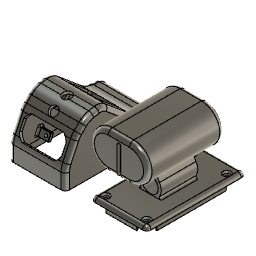
Boitier_CanneASon (Autodesk Fusion 360 design; units mm, degrees)
Autodesk Fusion 360 part; units mm, degrees
sketch "Sketch1" plane through (0, 0, 0) normal (1, 0, 0) x (0, 1, 0)
  line L0 (0, 0) -> (0, 12)
  line L1 (0, 12) -> (8.874983, 31.032464)
  line L2 (0, 12) -> (19, 12) construction
  line L3 (8.874983, 31.032464) -> (18.067372, 40.224852)
  line L4 (8.874983, 31.032464) -> (18.029747, 31.032464) construction
  line L5 (18.067372, 40.224852) -> (30.869872, 42.482278)
  line L6 (18.067372, 40.224852) -> (25.100815, 40.224852) construction
  line L7 (0, 0) -> (80, 0)
  line L8 (30.869872, 42.482278) -> (32.826168, 42.066455)
  line L9 (30.869872, 42.482278) -> (38.024636, 42.482278) construction
  line L10 (32.826168, 42.066455) -> (59.637723, 19.568888)
  line L11 (32.826168, 42.066455) -> (72.849817, 42.066455) construction
  line L12 (59.637723, 19.568888) -> (74.582285, 17.593812)
  line L13 (74.582285, 17.593812) -> (80, 0)
  dimension "d1" = 12
  dimension "d2" = 65
  dimension "d3" = 21
  dimension "d4" = 13
  dimension "d5" = 45
  dimension "d6" = 13
  dimension "d7" = 10
  dimension "d8" = 80
  dimension "d16" = 2
  dimension "d17" = 12
  dimension "d18" = 40
  dimension "d19" = 35
  constraint coincident L0.start L7.start
  constraint vertical L0
  constraint horizontal L2
  constraint horizontal L4
  constraint horizontal L6
  constraint perpendicular L0 L7
  constraint horizontal L9
  constraint horizontal L11
  measures "d1" distance of L0.start L0.end
  measures "d2" angle of L1 L2
  measures "d5" angle of L3 L4
  measures "d7" angle of L5 L6
  measures "d8" distance of L0.start L7.end
  measures "d17" angle of L8 L9
  measures "d18" angle of L10 L11
extrude "Extrude2" add sketch "Sketch1" along normal blind 46 contours L0 L1 L3 L5 L7 L8 L10 L12 L13 picked at (46.545908, 6.522963) makes body 1
sketch "Sketch2" plane through (0, -11.07874, 11.07874) normal (0, -0.707107, 0.707107) x (1, 0, 0)
  line L0 (0, 41.218826) -> (0, 28.218826)
  line L1 (0, 28.218826) -> (46, 28.218826)
  line L2 (46, 28.218826) -> (46, 41.218826)
  line L3 (46, 41.218826) -> (0, 41.218826)
  circle A0 centre (23, 34.718826) radius 3.75
  dimension "d26" = 7.5
  measures "d26" diameter of A0
shell "Shell2" thickness 2.5 removed faces 1 at (15.333333, 26.666667, 0) on bodies 1
extrude "Extrude3" cut sketch "Sketch2" against normal blind 15 contours A0 picked at (22.721849, 35.827351) bodies 1
sketch "Sketch3" plane through (0, -6.334057, 35.922221) normal (0, -0.173648, 0.984808) x (1, 0, 0)
  line L0 (0, 37.77786) -> (0, 24.77786)
  line L1 (0, 24.77786) -> (46, 24.77786)
  line L2 (46, 24.77786) -> (46, 37.77786)
  line L3 (46, 37.77786) -> (0, 37.77786)
  circle A0 centre (23, 31.27786) radius 3.75
  dimension "d30" = 7.5
  measures "d30" diameter of A0
extrude "Extrude4" cut sketch "Sketch3" against normal blind 6 contours A0 picked at (22.721849, 32.386384) bodies 1
sketch "Sketch7" plane through (0, 34.276667, 40.849341) normal (0, 0.642788, 0.766044) x (-1, 0, 0)
  line L0 (0, -33.106508) -> (0, 1.893492)
  line L1 (0, 1.893492) -> (-46, 1.893492)
  line L2 (-46, 1.893492) -> (-46, -33.106508)
  line L3 (-33.1, -28.248154) -> (-12.9, -28.248154)
  line L4 (-10.9, -26.248154) -> (-10.9, -6.048154)
  line L5 (-12.9, -4.048154) -> (-33.1, -4.048154)
  line L6 (-35.1, -6.048154) -> (-35.1, -26.248154)
  arc A0 (-33.1, -4.048154) -> (-35.1, -6.048154) centre (-33.1, -6.048154) ccw
  arc A1 (-35.1, -26.248154) -> (-33.1, -28.248154) centre (-33.1, -26.248154) ccw
  arc A2 (-12.9, -28.248154) -> (-10.9, -26.248154) centre (-12.9, -26.248154) ccw
  arc A3 (-10.9, -6.048154) -> (-12.9, -4.048154) centre (-12.9, -6.048154) ccw
  line L7 (-46, -33.106508) -> (0, -33.106508)
  point P0 (-35.1, -28.248154)
  point P1 (-10.9, -28.248154)
  point P2 (-35.1, -4.048154)
  dimension "d42" = 24.2
  dimension "d43" = 24.2
  dimension "d44" = 2
  constraint horizontal L3
  constraint vertical L4
  constraint horizontal L5
  constraint vertical L6
  constraint tangent L5 A0
  constraint tangent L6 A0
  constraint tangent L3 A1
  constraint tangent L6 A1
  constraint equal A0 A1
  constraint tangent L3 A2
  constraint tangent L4 A2
  constraint equal A0 A2
  constraint tangent L4 A3
  constraint tangent L5 A3
  constraint equal A0 A3
  measures "d44" radius of A0
extrude "Extrude7" add sketch "Sketch7" against normal blind 14 separate body contours L3 L4 L5 L6 A0 A1 A2 A3 picked at (-19.633333, -13.448154) makes body 2
shell "Shell3" thickness 3 outward yes removed faces 1 at (26.366667, 44.578551, 32.205034) on bodies 2
extrude "Extrude8" cut sketch "Sketch7" against normal blind 14 contours L3 L4 L5 L6 A0 A1 A2 A3 picked at (-19.633333, -13.448154) bodies 1
combine "Combine1" operation add target body 1 tool bodies 2
sketch "Sketch8" plane through (0, -4.596267, 2.143274) normal (0, -0.906308, 0.422618) x (1, 0, 0)
  line L0 (0, 31.875693) -> (0, 10.875693)
  line L1 (0, 10.875693) -> (46, 10.875693)
  line L2 (46, 10.875693) -> (46, 31.875693)
  line L3 (46, 31.875693) -> (0, 31.875693)
  line L4 (5.6, 12.175693) -> (40.4, 12.175693)
  line L5 (40.4, 12.175693) -> (40.4, 30.575693)
  line L6 (40.4, 30.575693) -> (5.6, 30.575693)
  line L7 (5.6, 30.575693) -> (5.6, 12.175693)
  line L8 (5.6, 12.175693) -> (5.6, 17.175693)
  line L9 (5.6, 21.375693) -> (15.6, 21.375693)
  circle A0 centre (15.6, 21.375693) radius 10.846197
  line L10 (40.4, 21.375693) -> (30.4, 21.375693)
  line L11 (40.4, 30.575693) -> (40.4, 25.575693)
  circle A1 centre (30.4, 21.375693) radius 10.846197
  dimension "d58" = 34.8
  dimension "d59" = 18.4
  dimension "d61" = 5
  dimension "d62" = 10
  dimension "d63" = 10
  dimension "d64" = 5
  constraint horizontal L4
  constraint vertical L5
  constraint horizontal L6
  constraint vertical L7
  constraint perpendicular L4 L8
  constraint perpendicular L7 L9
  constraint perpendicular L5 L10
  constraint perpendicular L6 L11
extrude "Extrude9" cut sketch "Sketch8" against normal blind 11 contours L4 L6 L7 A0 A1 | L6 A0 A1 | L4 A0 A1 | L4 L5 L6 A0 A1 | A0 A1 picked at (10.458254, 19.308066) picked at (22.825261, 30.046675) picked at (23.174739, 12.704712) picked at (35.518079, 19.084776) picked at (21.871346, 21.375693) bodies 1
sketch "Sketch12" plane through (0, 14.436197, -6.731709) normal (0, 0.906308, -0.422618) x (-1, 0, 0)
  line L0 (-36.144563, 30.575693) -> (-40.4, 30.575693)
  line L1 (-40.4, 30.575693) -> (-40.4, 25.575693)
  arc A0 (-36.144563, 30.575693) -> (-40.4, 25.575693) centre (-30.4, 21.375693) ccw
  line L2 (-34.000001, 30.125693) -> (-44.000001, 30.125693)
  line L3 (-44.000001, 30.125693) -> (-44.000001, 24.125693)
  line L4 (-44.000001, 24.125693) -> (-34.000001, 24.125693)
  line L5 (-34.000001, 24.125693) -> (-34.000001, 30.125693)
  circle A1 centre (-37.000001, 27.125693) radius 1.2
  dimension "d95" = 10
  dimension "d96" = 6
  dimension "d97" = 2.4
  constraint horizontal L2
  constraint vertical L3
  constraint horizontal L4
  constraint vertical L5
  measures "d97" diameter of A1
extrude "Extrude12" add sketch "Sketch12" along normal blind 2.5 separate body contours L1 A0 L2 L3 L4 L5 | L1 A0 L2 picked at (-42.8, 26.609027) picked at (-39.081529, 29.134109) makes body 3
sketch "Sketch13" plane through (0, 14.436197, -6.731709) normal (0, 0.906308, -0.422618) x (-1, 0, 0)
  line L0 (-9.855437, 12.175693) -> (-5.6, 12.175693)
  line L1 (-5.6, 12.175693) -> (-5.6, 17.175693)
  arc A0 (-9.855437, 12.175693) -> (-5.6, 17.175693) centre (-15.6, 21.375693) ccw
  line L2 (-12, 12.625693) -> (-2.5, 12.625693)
  line L3 (-2.5, 12.625693) -> (-2.5, 18.625693)
  line L4 (-2.5, 18.625693) -> (-12, 18.625693)
  line L5 (-12, 18.625693) -> (-12, 12.625693)
  circle A1 centre (-9, 15.625693) radius 1.2
  dimension "d104" = 6
  dimension "d105" = 2.4
  constraint horizontal L2
  constraint vertical L3
  constraint horizontal L4
  constraint vertical L5
  measures "d105" diameter of A1
extrude "Extrude13" add sketch "Sketch13" along normal blind 2.5 separate body contours L1 A0 L2 L3 L4 L5 | L1 A0 L2 picked at (-3.533333, 16.14236) picked at (-6.918471, 13.617278) makes body 4
fillet "Fillet8" radius 0.3 16 edges at (39.000001, 24.632155, 15.133595) (39.000001, 27.167865, 20.571441) (39.000001, 29.433635, 19.514896) (39.000001, 26.897925, 14.077049) (34.000001, 28.30075, 20.043169) (34.000001, 25.76504, 14.605322) (34.000001, 25.90001, 17.852518) (34.000001, 28.16578, 16.795972) (7.25, 22.307755, 10.148902) (7.25, 19.772045, 4.711055) (7.25, 24.573525, 9.092356) (7.25, 22.037815, 3.654509) (12, 23.44064, 9.620629) (12, 21.0399, 7.429978) (12, 20.90493, 4.182782) (12, 23.30567, 6.373433) on bodies 3 4
combine "Combine2" operation add target body 1 tool bodies 4 3
fillet "Fillet9" radius 1.5 8 edges at (2.5, 20.90493, 4.182782) (2.5, 19.888816, 4.753556) (2.5, 21.0399, 7.429978) (2.5, 22.350256, 10.032132) (2.5, 23.44064, 9.620629) (2.5, 24.456754, 9.049855) (2.5, 23.30567, 6.373433) (2.5, 21.995314, 3.77128) on bodies 1
fillet "Fillet10" radius 1.5 8 edges at (43.5, 28.16578, 16.795972) (43.5, 29.316865, 19.472395) (43.5, 28.30075, 20.043169) (43.5, 27.210366, 20.454671) (43.5, 25.90001, 17.852518) (43.5, 24.748926, 15.176095) (43.5, 25.76504, 14.605322) (43.5, 26.855424, 14.193819) on bodies 1
sketch "Sketch14" plane through (0, 25.277641, 30.124719) normal (0, 0.642788, 0.766044) x (-1, 0, 0)
  arc A0 (-10.9, -6.048154) -> (-12.9, -4.048154) centre (-12.9, -6.048154) ccw
  line L0 (-12.9, -4.048154) -> (-33.1, -4.048154)
  arc A1 (-33.1, -4.048154) -> (-35.1, -6.048154) centre (-33.1, -6.048154) ccw
  line L1 (-35.1, -6.048154) -> (-35.1, -26.248154)
  arc A2 (-35.1, -26.248154) -> (-33.1, -28.248154) centre (-33.1, -26.248154) ccw
  line L2 (-33.1, -28.248154) -> (-12.9, -28.248154)
  arc A3 (-12.9, -28.248154) -> (-10.9, -26.248154) centre (-12.9, -26.248154) ccw
  line L3 (-10.9, -26.248154) -> (-10.9, -6.048154)
  line L4 (-32.5, -28.248154) -> (-13.5, -28.248154)
  line L5 (-13.5, -28.248154) -> (-13.5, -3.748154)
  line L6 (-13.5, -3.748154) -> (-32.5, -3.748154)
  line L7 (-32.5, -3.748154) -> (-32.5, -28.248154)
  dimension "d115" = 19
  constraint horizontal L4
  constraint vertical L5
  constraint horizontal L6
  constraint vertical L7
extrude "Extrude14" cut sketch "Sketch14" against normal blind 2 contours L0 L2 L4 L5 L7 picked at (-26.166667, -12.11482) bodies 1
extrude "Extrude15" cut 1 faces at (26.166667, 33.272556, 20.805373) along direction (0, -0.64278761, -0.76604444) blind 1 on bodies 1 bodies 1
sketch "Sketch15" plane through (0, 23.937475, -20.085926) normal (0, 0.766044, -0.642788) x (-1, 0, 0)
  line L0 (-12.9, 50.825028) -> (-33.1, 50.825028)
  line L1 (-33.1, 50.825028) -> (-33.1, 36.325028)
  line L2 (-33.1, 36.325028) -> (-12.9, 36.325028)
  line L3 (-12.9, 36.325028) -> (-12.9, 50.825028)
  line L4 (-33.1, 36.325028) -> (-29.35, 36.325028)
  line L5 (-29.35, 36.325028) -> (-16.35, 36.325028)
  line L6 (-16.35, 36.325028) -> (-16.35, 50.825028)
  line L7 (-16.35, 50.825028) -> (-29.35, 50.825028)
  line L8 (-29.35, 50.825028) -> (-29.35, 36.325028)
  dimension "d120" = 3.75
  dimension "d121" = 13
  dimension "d122" = 14.5
  constraint perpendicular L1 L4
  constraint horizontal L5
  constraint vertical L6
  constraint horizontal L7
  constraint vertical L8
extrude "Extrude16" cut sketch "Sketch15" against normal blind 31 contours L0 L2 L5 L6 L7 L8 picked at (-20.683333, 41.158361) bodies 1
fillet "Fillet11" radius 2 4 edges at (29.35, 46.137686, 8.704841) (29.35, 25.301277, 26.188664) (16.35, 25.301277, 26.188664) (16.35, 46.137686, 8.704841) on bodies 1
sketch "Sketch20" plane through (43.5, 0, 0) normal (-1, 0, 0) x (0, -1, 0)
  line L0 (-77.384156, 0) -> (-2.5, 0)
  line L1 (-2.5, 0) -> (-2.5, 11.445763)
  line L2 (-2.5, 11.445763) -> (-10.954455, 29.576402)
  line L3 (-10.954455, 29.576402) -> (-19.277764, 37.89971)
  line L4 (-19.277764, 37.89971) -> (-30.825425, 39.935874)
  line L5 (-30.825425, 39.935874) -> (-31.696689, 39.750681)
  line L6 (-31.696689, 39.750681) -> (-58.58844, 17.185823)
  line L7 (-58.58844, 17.185823) -> (-72.664938, 15.32547)
  line L8 (-72.664938, 15.32547) -> (-77.384156, 0)
  line L9 (-28.384172, 13.715014) -> (-30.666311, 18.609076)
  arc A0 (-29.79567, 21.001143) -> (-30.666311, 18.609076) centre (-29.034957, 19.369789) ccw
  line L10 (-29.79567, 21.001143) -> (-28.073685, 21.804118)
  arc A1 (-25.681618, 20.933476) -> (-28.073685, 21.804118) centre (-27.312972, 20.172764) ccw
  line L11 (-25.681618, 20.933476) -> (-23.399479, 16.039414)
  arc A2 (-24.27012, 13.647348) -> (-23.399479, 16.039414) centre (-25.030833, 15.278702) ccw
  line L12 (-24.27012, 13.647348) -> (-25.992105, 12.844373)
  arc A3 (-28.384172, 13.715014) -> (-25.992105, 12.844373) centre (-26.752818, 14.475727) ccw
  line L13 (-71.626194, 13.560847) -> (-57.426194, 13.560847)
  line L14 (-57.426194, 13.560847) -> (-57.426194, 4.360847)
  line L15 (-57.426194, 4.360847) -> (-71.626194, 4.360847)
  line L16 (-71.626194, 4.360847) -> (-71.626194, 13.560847)
  dimension "d132" = 14.2
  dimension "d133" = 9.2
  constraint horizontal L13
  constraint vertical L14
  constraint horizontal L15
  constraint vertical L16
extrude "Extrude17" cut sketch "Sketch20" against normal blind 17 contours L13 L14 L15 L16 picked at (-66.892861, 10.494181) bodies 1
sketch "Sketch21" plane through (2.5, 0, 0) normal (1, 0, 0) x (0, 1, 0)
  line L0 (2.5, 0) -> (77.384156, 0)
  line L1 (77.384156, 0) -> (72.664938, 15.32547)
  line L2 (72.664938, 15.32547) -> (58.58844, 17.185823)
  line L3 (58.58844, 17.185823) -> (31.696689, 39.750681)
  line L4 (31.696689, 39.750681) -> (30.825425, 39.935874)
  line L5 (30.825425, 39.935874) -> (19.277764, 37.89971)
  line L6 (19.277764, 37.89971) -> (10.954455, 29.576402)
  line L7 (10.954455, 29.576402) -> (2.5, 11.445763)
  line L8 (2.5, 11.445763) -> (2.5, 0)
  line L9 (21.131995, 2.421833) -> (19.41001, 3.224808)
  arc A0 (18.539369, 5.616875) -> (19.41001, 3.224808) centre (20.170723, 4.856162) ccw
  line L10 (18.539369, 5.616875) -> (20.821508, 10.510937)
  arc A1 (23.213575, 11.381578) -> (20.821508, 10.510937) centre (22.452862, 9.750224) ccw
  line L11 (23.213575, 11.381578) -> (24.93556, 10.578603)
  arc A2 (25.806201, 8.186536) -> (24.93556, 10.578603) centre (24.174847, 8.947249) ccw
  line L12 (25.806201, 8.186536) -> (23.524062, 3.292474)
  arc A3 (21.131995, 2.421833) -> (23.524062, 3.292474) centre (21.892708, 4.053187) ccw
  line L13 (26, 0) -> (17, 0)
  line L14 (17, 0) -> (17, 4)
  line L15 (17, 4) -> (26, 4)
  line L16 (26, 4) -> (26, 0)
  dimension "d136" = 4
  constraint horizontal L13
  constraint vertical L14
  constraint horizontal L15
  constraint vertical L16
  constraint coincident L0 L13.start
  measures "d136" distance of L13.start L15.end
extrude "Extrude18" cut sketch "Sketch21" along normal blind 12 contours L0 L9 A0 L12 A3 L13 L14 L15 L16 | L9 A0 L12 A3 L15 picked at (21.626143, 0.751081) picked at (21.465331, 3.215547) bodies 1
sketch "Sketch23" plane through (46, 0, 0) normal (1, 0, 0) x (0, 1, 0)
  line L0 (57.426194, 4.360847) -> (57.426194, 13.560847)
  line L1 (57.426194, 13.560847) -> (71.626194, 13.560847)
  line L2 (71.626194, 13.560847) -> (71.626194, 4.360847)
  line L3 (71.626194, 4.360847) -> (57.426194, 4.360847)
  line L4 (0, 0) -> (80, 0)
  line L5 (80, 0) -> (74.582285, 17.593812)
  line L6 (74.582285, 17.593812) -> (59.637723, 19.568888)
  line L7 (59.637723, 19.568888) -> (32.826168, 42.066455)
  line L8 (32.826168, 42.066455) -> (30.869872, 42.482278)
  line L9 (30.869872, 42.482278) -> (18.067372, 40.224852)
  line L10 (18.067372, 40.224852) -> (8.874983, 31.032464)
  line L11 (8.874983, 31.032464) -> (0, 12)
  line L12 (0, 12) -> (0, 0)
  line L13 (0, 0) -> (0, -4)
  line L14 (0, -4) -> (97.000001, -4)
  line L15 (80, 0) -> (81.231732, -4)
  dimension "d143" = 4
  constraint coincident L4.start L12.end
  constraint perpendicular L4 L13
  constraint perpendicular L13 L14
  constraint coincident L4.end L5.start
  constraint parallel L5 L15
  measures "d143" distance of L4.start L13.end
extrude "Extrude20" add sketch "Sketch23" against normal blind 46 separate body contours L4 L13 L14 L15 picked at (53.743911, -2.666667) makes body 5
shell "Shell4" thickness 2.5 removed faces 2 at (30.666667, 27.077244, -4) at (30.666667, 26.666667, 0) on bodies 5
combine "Combine3" operation add target body 1 tool bodies 5
move_body "Move1" bodies 1 to x (1, 0, 0) y (0, 1, 0) z (0, 0, 1) at (0, 0, 4)
sketch "Sketch24" plane through (0, 0, 0) normal (0, 0, -1) x (1, 0, 0)
  line L0 (2.5, -2.5) -> (43.5, -2.5)
  line L1 (43.5, -2.5) -> (43.5, -78.615887)
  line L2 (43.5, -78.615887) -> (2.5, -78.615887)
  line L3 (2.5, -78.615887) -> (2.5, -2.5)
  line L4 (46, -81.231732) -> (46, 0)
  line L5 (46, 0) -> (0, 0)
  line L6 (0, 0) -> (0, -81.231732)
  line L7 (0, -81.231732) -> (46, -81.231732)
  line L8 (0, 0) -> (46, 0)
  line L9 (46, 0) -> (46, -81.231732)
  line L10 (46, -81.231732) -> (0, -81.231732)
  line L11 (0, -81.231732) -> (0, 0)
  constraint horizontal L8
  constraint vertical L9
  constraint horizontal L10
  constraint vertical L11
  constraint coincident L5.end L6.start
move_body "Move2" bodies 1 to x (1, 0, 0) y (0, 1, 0) z (0, 0, 1) at (-65, 0, 0)
extrude "Extrude21" add sketch "Sketch24" against normal blind 3 separate body contours L0 L1 L2 L3 | L4 L5 L6 L7 L8 L9 L10 L11 picked at (16.166667, -27.871962) picked at (29.833333, -80.359784) makes body 6
sketch "Sketch25" plane through (0, 0, 3) normal (0, 0, 1) x (-1, 0, 0)
  line L0 (-46, -81.231732) -> (0, -81.231732)
  line L1 (0, -81.231732) -> (0, 0)
  line L2 (0, 0) -> (-46, 0)
  line L3 (-46, 0) -> (-46, -81.231732)
  line L4 (-2.95, -69.1) -> (-2.05, -69.1)
  line L5 (-2.05, -69.1) -> (-2.05, -2.05)
  line L6 (-2.05, -2.05) -> (-43.95, -2.05)
  line L7 (-43.95, -2.05) -> (-43.95, -69.100001)
  line L8 (-43.95, -69.100001) -> (-43.05, -69.100001)
  line L9 (-43.05, -69.100001) -> (-43.05, -2.950001)
  line L10 (-43.05, -2.950001) -> (-2.95, -2.950001)
  line L11 (-2.95, -69.1) -> (-2.95, -2.950001)
  dimension "d151" = 0.9
  dimension "d152" = 67.05
  dimension "d153" = 41.9
  dimension "d154" = 67.050001
  dimension "d155" = 0.9
  dimension "d156" = 66.15
  dimension "d158" = 40.1
  constraint perpendicular L4 L5
  constraint perpendicular L3 L6
  constraint perpendicular L6 L7
  constraint perpendicular L7 L8
  constraint perpendicular L8 L9
  constraint perpendicular L9 L10
  constraint perpendicular L10 L11
  measures "d151" distance of L4.start L4.end
  measures "d152" distance of L4.end L5.end
  measures "d153" distance of L6.end L5.end
extrude "Extrude22" add sketch "Sketch25" along normal blind 5 contours L4 L5 L6 L7 L8 L9 L10 L11 picked at (-43.65, -24.700001) bodies 6
sketch "Sketch27" plane through (0, 0, 0) normal (0, 0, -1) x (1, 0, 0)
  line L0 (-62.5, -2.5) -> (-21.5, -2.5)
  line L1 (-21.5, -2.5) -> (-21.5, -78.615887)
  line L2 (-21.5, -78.615887) -> (-62.5, -78.615887)
  line L3 (-62.5, -78.615887) -> (-62.5, -2.5)
  line L4 (-19, -81.231732) -> (-19, 0)
  line L5 (-19, 0) -> (-65, 0)
  line L6 (-65, 0) -> (-65, -81.231732)
  line L7 (-65, -81.231732) -> (-19, -81.231732)
  line L8 (-63.05, -1.95) -> (-63.05, -74.1)
  line L9 (-63.05, -1.95) -> (-20.95, -1.95)
  line L10 (-20.95, -1.95) -> (-20.95, -74.1)
  line L11 (-20.95, -74.1) -> (-21.5, -74.1)
  line L12 (-21.5, -2.5) -> (-62.5, -2.5)
  line L13 (-63.05, -74.1) -> (-62.5, -74.1)
  line L14 (-62.5, -2.5) -> (-62.5, -74.1)
  dimension "d168" = 72.15
  dimension "d169" = 42.1
  dimension "d170" = 72.15
  constraint perpendicular L0 L8
  constraint perpendicular L4 L9
  constraint perpendicular L9 L10
  constraint coincident L1 L11.end
  constraint perpendicular L1 L11
  constraint coincident L0.end L1.start
  constraint coincident L0.start L3.end
  constraint coincident L3 L13.end
  constraint perpendicular L3 L13
  measures "d168" distance of L8.start L8.end
  measures "d169" distance of L8.start L9.end
  measures "d170" distance of L9.end L10.end
extrude "Extrude23" cut sketch "Sketch27" against normal blind 5.3 contours L0 L1 L3 L8 L9 L10 L11 L12 L13 L14 picked at (-21.133333, -26.183333) bodies 1
sketch "Sketch28" plane through (0, 0, 3) normal (0, 0, 1) x (-1, 0, 0)
  line L0 (-2.95, -69.1) -> (-2.95, -2.950001)
  line L1 (-2.95, -2.950001) -> (-43.05, -2.950001)
  line L2 (-43.05, -2.950001) -> (-43.05, -69.100001)
  line L3 (-43.95, -69.100001) -> (-43.95, -2.05)
  line L4 (-43.95, -2.05) -> (-2.05, -2.05)
  line L5 (-2.05, -2.05) -> (-2.05, -69.1)
  line L6 (-46, -81.231732) -> (0, -81.231732)
  line L7 (0, -81.231732) -> (0, 0)
  line L8 (0, 0) -> (-46, 0)
  line L9 (-46, 0) -> (-46, -81.231732)
  line L10 (-2.05, -2.05) -> (-10.05, -2.05)
  line L11 (-10.05, -2.05) -> (-10.05, -10.05)
  line L12 (-10.05, -10.05) -> (-2.05, -10.05)
  line L13 (-2.05, -10.05) -> (-2.05, -2.05)
  line L14 (-43.95, -2.05) -> (-35.95, -2.05)
  line L15 (-35.95, -2.05) -> (-35.95, -10.05)
  line L16 (-35.95, -10.05) -> (-43.95, -10.05)
  line L17 (-43.95, -10.05) -> (-43.95, -2.05)
  line L18 (-2.05, -69.1) -> (-2.95, -69.1)
  line L19 (-43.05, -69.100001) -> (-43.95, -69.100001)
  dimension "d174" = 8
  dimension "d175" = 8
  dimension "d176" = 8
  dimension "d177" = 8
  constraint horizontal L10
  constraint vertical L11
  constraint horizontal L12
  constraint vertical L13
  constraint coincident L4.end L5.start
  constraint horizontal L14
  constraint vertical L15
  constraint horizontal L16
  constraint vertical L17
  constraint coincident L3.end L4.start
  measures "d174" distance of L4.end L10.end
  measures "d175" distance of L4.end L12.end
  measures "d176" distance of L3.end L14.end
  measures "d177" distance of L3.end L16.end
extrude "Extrude24" add sketch "Sketch28" along normal blind 1 contours L0 L1 L11 L12 | L1 L2 L15 L16 picked at (-7.683333, -7.683334) picked at (-40.683333, -5.316667) bodies 6
sketch "Sketch29" plane through (0, 0, 0) normal (0, 0, -1) x (1, 0, 0)
  line L0 (-19, -81.231732) -> (-19, 0)
  line L1 (-19, 0) -> (-65, 0)
  line L2 (-65, 0) -> (-65, -81.231732)
  line L3 (-65, -81.231732) -> (-19, -81.231732)
  line L4 (-62.5, -74.1) -> (-63.05, -74.1)
  line L5 (-63.05, -74.1) -> (-63.05, -1.95)
  line L6 (-63.05, -1.95) -> (-20.95, -1.95)
  line L7 (-20.95, -1.95) -> (-20.95, -74.1)
  line L8 (-20.95, -74.1) -> (-21.5, -74.1)
  line L9 (-21.5, -74.1) -> (-21.5, -78.615887)
  line L10 (-21.5, -78.615887) -> (-62.5, -78.615887)
  line L11 (-62.5, -78.615887) -> (-62.5, -74.1)
  line L12 (-63.05, -1.95) -> (-54.95, -1.95)
  line L13 (-54.95, -1.95) -> (-54.95, -10.05)
  line L14 (-54.95, -10.05) -> (-63.05, -10.05)
  line L15 (-63.05, -10.05) -> (-63.05, -1.95)
  line L16 (-20.95, -1.95) -> (-29.05, -1.95)
  line L17 (-29.05, -1.95) -> (-29.05, -10.05)
  line L18 (-29.05, -10.05) -> (-20.95, -10.05)
  line L19 (-20.95, -10.05) -> (-20.95, -1.95)
  dimension "d180" = 8.1
  dimension "d181" = 8.1
  dimension "d182" = 8.1
  dimension "d183" = 8.1
  constraint horizontal L12
  constraint vertical L13
  constraint horizontal L14
  constraint vertical L15
  constraint coincident L5.end L6.start
  constraint horizontal L16
  constraint vertical L17
  constraint horizontal L18
  constraint vertical L19
  constraint coincident L6.end L7.start
  measures "d180" distance of L5.end L12.end
  measures "d181" distance of L5.end L14.end
  measures "d182" distance of L6.end L16.end
  measures "d183" distance of L6.end L18.end
extrude "Extrude25" add sketch "Sketch29" against normal blind 6 contours L5 L6 L12 L13 L14 L15 | L6 L7 L16 L17 L18 L19 picked at (-60.35, -4.65) picked at (-26.35, -4.65) bodies 1
extrude "Extrude26" cut sketch "Sketch29" against normal blind 1 contours L5 L6 L12 L13 L14 L15 | L6 L7 L16 L17 L18 L19 picked at (-60.35, -4.65) picked at (-26.35, -4.65) bodies 1
sketch "Sketch30" plane through (0, 0, 1) normal (0, 0, -1) x (1, 0, 0)
  line L0 (-63.05, -10.05) -> (-54.95, -10.05)
  line L1 (-54.95, -10.05) -> (-54.95, -1.95)
  line L2 (-54.95, -1.95) -> (-63.05, -1.95)
  line L3 (-63.05, -1.95) -> (-63.05, -10.05)
  line L4 (-63.05, -10.05) -> (-63.05, -67.55)
  line L5 (-63.05, -67.55) -> (-54.95, -67.55)
  line L6 (-54.95, -67.55) -> (-54.95, -76.15)
  line L7 (-54.95, -76.15) -> (-63.05, -76.15)
  line L8 (-63.05, -76.15) -> (-63.05, -67.55)
  line L9 (-20.95, -10.05) -> (-20.95, -67.55)
  line L10 (-20.95, -67.55) -> (-29.05, -67.55)
  line L11 (-29.05, -67.55) -> (-29.05, -76.15)
  line L12 (-29.05, -76.15) -> (-20.95, -76.15)
  line L13 (-20.95, -76.15) -> (-20.95, -67.55)
  dimension "d188" = 57.5
  dimension "d189" = 8.1
  dimension "d190" = 8.6
  dimension "d196" = 57.5
  dimension "d197" = 8.1
  dimension "d198" = 8.6
  constraint coincident L0.start L3.end
  constraint perpendicular L0 L4
  constraint horizontal L5
  constraint vertical L6
  constraint horizontal L7
  constraint vertical L8
  constraint vertical L9
  constraint horizontal L10
  constraint vertical L11
  constraint horizontal L12
  constraint vertical L13
  measures "d188" distance of L0.start L4.end
  measures "d189" distance of L4.end L5.end
  measures "d190" distance of L4.end L7.end
  measures "d196" distance of L9.start L9.end
  measures "d197" distance of L9.end L10.end
  measures "d198" distance of L9.end L12.end
extrude "Extrude28" add sketch "Sketch30" against normal blind 5 contours L5 L6 L7 L8 | L10 L11 L12 L13 picked at (-57.65, -70.416667) picked at (-26.35, -70.416667) bodies 1
extrude "Extrude29" cut 2 faces at (-21.316667, 74.1, 0.666667) (-62.866667, 74.1, 0.333333) along direction (0, 1, 0) blind 4 on bodies 1 bodies 1
sketch "Sketch31" plane through (0, 0, 8) normal (0, 0, 1) x (-1, 0, 0)
  line L0 (-2.05, -69.1) -> (-2.05, -2.05)
  line L1 (-2.05, -2.05) -> (-43.95, -2.05)
  line L2 (-43.95, -2.05) -> (-43.95, -69.100001)
  line L3 (-43.95, -69.100001) -> (-43.05, -69.100001)
  line L4 (-43.05, -69.100001) -> (-43.05, -2.950001)
  line L5 (-43.05, -2.950001) -> (-2.95, -2.950001)
  line L6 (-2.95, -2.950001) -> (-2.95, -69.1)
  line L7 (-2.95, -69.1) -> (-2.05, -69.1)
  line L8 (-2.05, -2.05) -> (-2.05, -10.35)
  line L9 (-2.05, -10.35) -> (-2.95, -10.35)
  line L10 (-2.05, -2.05) -> (-10.35, -2.05)
  line L11 (-10.35, -2.05) -> (-10.35, -2.950001)
  line L12 (-10.35, -2.950001) -> (-2.95, -2.950001)
  line L13 (-2.95, -2.950001) -> (-2.95, -10.35)
  line L14 (-43.95, -2.05) -> (-43.95, -10.35)
  line L15 (-43.95, -10.35) -> (-43.05, -10.35)
  line L16 (-43.95, -2.05) -> (-35.65, -2.05)
  line L17 (-35.65, -2.05) -> (-35.65, -2.950001)
  line L18 (-35.65, -2.950001) -> (-43.05, -2.950001)
  line L19 (-43.05, -10.35) -> (-43.05, -2.950001)
  dimension "d203" = 8.3
  dimension "d204" = 8.3
  dimension "d205" = 8.3
  dimension "d206" = 8.3
  constraint coincident L0.end L1.start
  constraint perpendicular L1 L8
  constraint coincident L6 L9.end
  constraint perpendicular L6 L9
  constraint perpendicular L0 L10
  constraint perpendicular L5 L11
  constraint coincident L1.end L2.start
  constraint perpendicular L1 L14
  constraint coincident L4 L15.end
  constraint perpendicular L4 L15
  constraint perpendicular L2 L16
  constraint perpendicular L5 L17
  measures "d203" distance of L0.end L8.end
  measures "d204" distance of L0.end L10.end
  measures "d205" distance of L1.end L14.end
  measures "d206" distance of L1.end L16.end
extrude "Extrude30" cut sketch "Sketch31" against normal blind 4 contours L0 L1 L5 L6 L8 L9 L10 L11 L12 L13 | L1 L2 L4 L5 L14 L15 L16 L17 L18 L19 picked at (-5.116667, -2.35) picked at (-40.883333, -2.35) bodies 6
sketch "Sketch32" plane through (0, 0, 3) normal (0, 0, 1) x (-1, 0, 0)
  line L0 (-35.95, -10.05) -> (-43.05, -10.05)
  line L1 (-43.05, -10.05) -> (-43.05, -69.100001)
  line L2 (-43.05, -69.100001) -> (-43.95, -69.100001)
  line L3 (-43.95, -69.100001) -> (-43.95, -2.05)
  line L4 (-43.95, -2.05) -> (-2.05, -2.05)
  line L5 (-2.05, -2.05) -> (-2.05, -69.1)
  line L6 (-2.05, -69.1) -> (-2.95, -69.1)
  line L7 (-2.95, -69.1) -> (-2.95, -10.05)
  line L8 (-2.95, -10.05) -> (-10.05, -10.05)
  line L9 (-10.05, -10.05) -> (-10.05, -2.950001)
  line L10 (-10.05, -2.950001) -> (-35.95, -2.950001)
  line L11 (-35.95, -2.950001) -> (-35.95, -10.05)
  line L12 (-46, -81.231732) -> (0, -81.231732)
  line L13 (0, -81.231732) -> (0, 0)
  line L14 (0, 0) -> (-46, 0)
  line L15 (-46, 0) -> (-46, -81.231732)
  line L16 (-2.95, -10.05) -> (-2.95, -67.55)
  line L17 (-2.95, -67.55) -> (-2.05, -67.55)
  line L18 (-2.05, -67.55) -> (-10.05, -67.55)
  line L19 (-10.05, -67.55) -> (-10.05, -76.15)
  line L20 (-10.05, -76.15) -> (-2.05, -76.15)
  line L21 (-2.05, -76.15) -> (-2.05, -67.55)
  line L22 (-43.05, -10.05) -> (-43.05, -67.55)
  line L23 (-43.05, -67.55) -> (-43.95, -67.55)
  line L24 (-43.95, -67.55) -> (-35.95, -67.55)
  line L25 (-35.95, -67.55) -> (-35.95, -76.15)
  line L26 (-35.95, -76.15) -> (-43.95, -76.15)
  line L27 (-43.95, -76.15) -> (-43.95, -67.55)
  dimension "d211" = 57.5
  dimension "d212" = 8
  dimension "d213" = 8.6
  dimension "d214" = 57.5
  dimension "d215" = 8
  dimension "d216" = 8.6
  constraint coincident L7.end L8.start
  constraint perpendicular L8 L16
  constraint coincident L5 L17.end
  constraint perpendicular L5 L17
  constraint horizontal L18
  constraint vertical L19
  constraint horizontal L20
  constraint vertical L21
  constraint coincident L0.end L1.start
  constraint perpendicular L0 L22
  constraint coincident L3 L23.end
  constraint perpendicular L3 L23
  constraint horizontal L24
  constraint vertical L25
  constraint horizontal L26
  constraint vertical L27
  measures "d211" distance of L7.end L16.end
  measures "d212" distance of L17.end L18.end
  measures "d213" distance of L17.end L20.end
  measures "d214" distance of L0.end L22.end
  measures "d215" distance of L23.end L24.end
  measures "d216" distance of L23.end L26.end
extrude "Extrude31" cut sketch "Sketch32" along normal blind 5 contours L1 L2 L3 L23 L24 L27 | L5 L6 L7 L17 L18 L21 picked at (-43.35, -68.066667) picked at (-2.35, -68.583333) bodies 6
extrude "Extrude32" add sketch "Sketch32" along normal blind 1 contours L1 L2 L24 L25 L26 L27 | L1 L2 L3 L23 L24 L27 | L5 L6 L7 L17 L18 L21 | L6 L7 L18 L19 L20 L21 picked at (-38.316667, -70.933334) picked at (-43.35, -68.066667) picked at (-2.35, -68.583333) picked at (-7.683333, -70.933333) bodies 6
extrude "Extrude39" cut 2 faces at (2.65, 67.55, 5.333333) (43.35, 67.55, 5.333333) along direction (0, -1, 0) blind 0.3 on bodies 6 bodies 6
sketch "Sketch37" plane through (0, 0, 4) normal (0, 0, 1) x (-1, 0, 0)
  line L0 (-35.95, -2.950001) -> (-35.65, -2.950001)
  line L1 (-35.65, -2.950001) -> (-35.65, -2.05)
  line L2 (-35.65, -2.05) -> (-43.95, -2.05)
  line L3 (-43.95, -2.05) -> (-43.95, -10.35)
  line L4 (-43.95, -10.35) -> (-43.05, -10.35)
  line L5 (-43.05, -10.35) -> (-43.05, -10.05)
  line L6 (-43.05, -10.05) -> (-35.95, -10.05)
  line L7 (-35.95, -10.05) -> (-35.95, -2.950001)
  line L8 (-10.05, -10.05) -> (-10.05, -6.05)
  line L9 (-10.05, -6.05) -> (-6.05, -6.05)
  circle A0 centre (-6.05, -6.05) radius 1.55
  line L10 (-35.95, -10.05) -> (-35.95, -6.05)
  line L11 (-35.95, -6.05) -> (-39.95, -6.05)
  circle A1 centre (-39.95, -6.05) radius 1.55
  line L12 (-10.05, -67.549998) -> (-6.05, -67.549998)
  line L13 (-6.05, -67.549998) -> (-6.05, -71.849998)
  circle A2 centre (-6.05, -71.849998) radius 1.55
  line L14 (-35.949999, -67.549998) -> (-39.949999, -67.549998)
  line L15 (-39.949999, -67.549998) -> (-39.949999, -71.849998)
  circle A3 centre (-39.949999, -71.849998) radius 1.55
  dimension "d263" = 4
  dimension "d264" = 4
  dimension "d265" = 3.1
  dimension "d266" = 4
  dimension "d267" = 4
  dimension "d268" = 3.1
  dimension "d269" = 4
  dimension "d270" = 4.3
  dimension "d271" = 3.1
  dimension "d272" = 4
  dimension "d273" = 4.3
  dimension "d274" = 3.1
  constraint vertical L8
  constraint perpendicular L8 L9
  constraint coincident L9.end A0.centre
  constraint coincident L6.end L7.start
  constraint perpendicular L6 L10
  constraint perpendicular L7 L11
  constraint coincident L11.end A1.centre
  constraint horizontal L12
  constraint perpendicular L12 L13
  constraint horizontal L14
  constraint perpendicular L14 L15
  measures "d263" distance of L8.start L8.end
  measures "d264" distance of L8.end L9.end
  measures "d265" diameter of A0
  measures "d266" distance of L6.end L10.end
  measures "d267" distance of L10.end L11.end
  measures "d268" diameter of A1
  measures "d271" diameter of A2
  measures "d274" diameter of A3
extrude "Extrude40" cut sketch "Sketch37" against normal blind 4 contours A0 | A1 | A2 | A3 picked at (-6.648466, -5.630802) picked at (-40.349357, -6.453946) picked at (-5.720026, -71.412863) picked at (-40.000154, -72.35425) bodies 6
sketch "Sketch38" plane through (0, 0, 1) normal (0, 0, -1) x (1, 0, 0)
  line L0 (-63.05, -67.55) -> (-63.05, -78.1)
  line L1 (-63.05, -78.1) -> (-62.5, -78.1)
  line L2 (-62.5, -78.1) -> (-62.5, -76.15)
  line L3 (-62.5, -76.15) -> (-54.95, -76.15)
  line L4 (-54.95, -76.15) -> (-54.95, -67.55)
  line L5 (-54.95, -67.55) -> (-63.05, -67.55)
  line L6 (-54.95, -67.55) -> (-58.95, -67.55)
  line L7 (-58.95, -67.55) -> (-58.95, -71.85)
  circle A0 centre (-58.808556, -71.85) radius 1.55
  line L8 (-29.050001, -67.550003) -> (-25.050001, -67.550003)
  line L9 (-25.050001, -67.550003) -> (-25.050001, -71.850003)
  circle A1 centre (-25.050001, -71.850003) radius 1.55
  line L10 (-54.949999, -10.05) -> (-58.949999, -10.05)
  line L11 (-58.949999, -10.05) -> (-58.949999, -6.05)
  circle A2 centre (-58.949999, -6.05) radius 1.55
  line L12 (-29.050001, -10.05) -> (-25.050001, -10.05)
  line L13 (-25.050001, -10.05) -> (-25.050001, -6.05)
  circle A3 centre (-25.050001, -6.05) radius 1.55
  dimension "d277" = 4
  dimension "d278" = 4.3
  dimension "d279" = 3.1
  dimension "d280" = 4
  dimension "d281" = 4.3
  dimension "d282" = 3.1
  dimension "d283" = 4
  dimension "d284" = 4
  dimension "d285" = 3.1
  dimension "d286" = 4
  dimension "d287" = 4
  dimension "d288" = 3.1
  constraint coincident L4.end L5.start
  constraint perpendicular L4 L6
  constraint perpendicular L3 L7
  constraint horizontal L8
  constraint perpendicular L8 L9
  constraint horizontal L10
  constraint perpendicular L10 L11
  constraint horizontal L12
  constraint perpendicular L12 L13
  measures "d277" distance of L4.end L6.end
  measures "d278" distance of L6.end L7.end
  measures "d279" diameter of A0
  measures "d282" diameter of A1
  measures "d285" diameter of A2
  measures "d288" diameter of A3
extrude "Extrude41" cut sketch "Sketch38" against normal blind 5 contours A0 | A1 | A2 | A3 picked at (-58.875765, -71.397717) picked at (-24.795839, -71.41846) picked at (-58.571587, -5.653099) picked at (-26.278356, -6.042135) bodies 1
sketch "Sketch39" plane through (0, 0, 0) normal (0, 0, -1) x (1, 0, 0)
  circle A0 centre (39.95, -6.05) radius 1.55
  circle A1 centre (6.05, -71.849998) radius 1.55
  circle A2 centre (6.05, -6.05) radius 1.55
  circle A3 centre (39.949999, -71.849998) radius 1.55
  line L0 (0, -81.231732) -> (46, -81.231732)
  line L1 (46, -81.231732) -> (46, 0)
  line L2 (46, 0) -> (0, 0)
  line L3 (0, 0) -> (0, -81.231732)
  circle A4 centre (6.05, -6.05) radius 3.25
  circle A5 centre (39.95, -6.05) radius 3.25
  circle A6 centre (6.05, -71.849998) radius 3.25
  circle A7 centre (39.949999, -71.849998) radius 3.25
  dimension "d291" = 6.5
  dimension "d292" = 6.5
  dimension "d293" = 6.5
  dimension "d294" = 6.5
  constraint concentric A2 A4
  constraint concentric A0 A5
  constraint concentric A1 A6
  constraint concentric A3 A7
  measures "d291" diameter of A4
  measures "d292" diameter of A5
  measures "d293" diameter of A6
  measures "d294" diameter of A7
extrude "Extrude42" cut sketch "Sketch39" against normal blind 2.2 contours A4 | A5 | A6 | A7 picked at (8.715462, -6.288468) picked at (42.615463, -6.288468) picked at (8.721233, -72.011461) picked at (42.615462, -72.088466) bodies 6
sketch "Sketch40" plane through (0, 0, 1) normal (0, 0, -1) x (1, 0, 0)
  circle A0 centre (-58.808556, -71.85) radius 1.55
  line L0 (-63.05, -67.55) -> (-63.05, -78.1)
  line L1 (-63.05, -78.1) -> (-62.5, -78.1)
  line L2 (-62.5, -78.1) -> (-62.5, -76.15)
  line L3 (-62.5, -76.15) -> (-54.95, -76.15)
  line L4 (-54.95, -76.15) -> (-54.95, -67.55)
  line L5 (-54.95, -67.55) -> (-63.05, -67.55)
  circle A1 centre (-58.808556, -71.85) radius 2.6
  dimension "d297" = 5.2
  constraint concentric A0 A1
  measures "d297" diameter of A1
sketch "Sketch41" plane through (0, 0, 1) normal (0, 0, -1) x (1, 0, 0)
  circle A0 centre (-25.050001, -71.850003) radius 1.55
  line L0 (-20.95, -78.1) -> (-20.95, -67.55)
  line L1 (-20.95, -67.55) -> (-29.05, -67.55)
  line L2 (-29.05, -67.55) -> (-29.05, -76.15)
  line L3 (-29.05, -76.15) -> (-21.5, -76.15)
  line L4 (-21.5, -76.15) -> (-21.5, -78.1)
  line L5 (-21.5, -78.1) -> (-20.95, -78.1)
  circle A1 centre (-25.050001, -71.850003) radius 2.6
  dimension "d298" = 5.2
  constraint concentric A0 A1
  measures "d298" diameter of A1
sketch "Sketch42" plane through (0, 0, 1) normal (0, 0, -1) x (1, 0, 0)
  circle A0 centre (-58.949999, -6.05) radius 1.55
  line L0 (-63.05, -10.05) -> (-54.95, -10.05)
  line L1 (-54.95, -10.05) -> (-54.95, -1.95)
  line L2 (-54.95, -1.95) -> (-63.05, -1.95)
  line L3 (-63.05, -1.95) -> (-63.05, -10.05)
  circle A1 centre (-58.949999, -6.05) radius 2.6
  dimension "d299" = 5.2
  constraint concentric A0 A1
  measures "d299" diameter of A1
sketch "Sketch43" plane through (0, 0, 1) normal (0, 0, -1) x (1, 0, 0)
  circle A0 centre (-25.050001, -6.05) radius 1.55
  line L0 (-20.95, -10.05) -> (-20.95, -1.95)
  line L1 (-20.95, -1.95) -> (-29.05, -1.95)
  line L2 (-29.05, -1.95) -> (-29.05, -10.05)
  line L3 (-29.05, -10.05) -> (-20.95, -10.05)
  circle A1 centre (-25.050001, -6.05) radius 2.6
  dimension "d300" = 5.2
  constraint concentric A0 A1
  measures "d300" diameter of A1
extrude "Extrude43" cut sketch "Sketch40" sketch "Sketch43" sketch "Sketch42" sketch "Sketch41" against normal blind 3 contours A1 picked at (-56.629693, -71.313085) of sketch 2 contours A1 picked at (-22.815452, -6.256176) of sketch 3 contours A1 picked at (-56.715449, -6.256175) of sketch 4 contours A1 picked at (-27.124505, -70.994343) bodies 1
fillet "Fillet12" radius 1.5 12 edges at (-54.95, 10.05, 3.5) (-29.05, 10.05, 3.5) (-54.95, 76.15, 3.5) (-54.95, 67.55, 3.5) (-29.05, 76.15, 3.5) (-29.05, 67.55, 3.5) (10.05, 76.15, 3.5) (10.05, 67.55, 3.5) (10.05, 10.05, 3.5) (35.95, 10.05, 3.5) (35.95, 67.55, 3.5) (35.95, 76.15, 3.5) on bodies 1 6
sketch "Sketch44" plane through (0, 0, 0) normal (0, 0, 1) x (1, 0, 0)
  circle A0 centre (125.000002, 45.000001) radius 6.65
  circle A1 centre (125.000002, 45.000001) radius 9.15
  line L0 (126.500002, 35.973789) -> (126.500002, 38.521382)
  line L1 (123.500002, 35.973789) -> (123.500002, 38.521382)
  line L2 (123.500002, 35.973789) -> (123.500002, 27.973789)
  line L3 (126.500002, 35.973789) -> (126.500002, 27.973789)
  line L4 (123.500002, 27.973789) -> (119.500002, 27.973789)
  line L5 (119.500002, 27.973789) -> (119.500002, 37.687511)
  line L6 (126.500002, 27.973789) -> (130.500002, 27.973789)
  line L7 (130.500002, 27.973789) -> (130.500002, 37.687511)
  dimension "d305" = 13.3
  dimension "d306" = 18.3
  dimension "d309" = 8
  dimension "d310" = 8
  dimension "d312" = 4
  constraint concentric A0 A1
  constraint parallel L1 L2
  constraint parallel L0 L3
  constraint perpendicular L2 L4
  constraint perpendicular L4 L5
  constraint perpendicular L3 L6
  constraint perpendicular L6 L7
  measures "d305" diameter of A0
  measures "d306" diameter of A1
extrude "Extrude44" add sketch "Sketch44" along normal blind 30 separate body contours A0 A1 L0 L1 | A1 L2 L4 L5 | A1 L3 L6 L7 picked at (118.147358, 49.684116) picked at (121.809942, 30.721989) picked at (128.190061, 30.721989) makes body 7
sketch "Sketch45" plane through (130.500002, 0, 0) normal (1, 0, 0) x (0, 1, 0)
  line L0 (27.973789, 0) -> (37.687511, 0)
  line L1 (37.687511, 0) -> (37.687511, 30)
  line L2 (37.687511, 30) -> (27.973789, 30)
  line L3 (27.973789, 30) -> (27.973789, 0)
  line L4 (27.973789, 30) -> (32.373789, 30)
  line L5 (32.373789, 30) -> (32.373789, 22)
  line L6 (32.373789, 22) -> (32.373789, 8)
  circle A0 centre (32.373789, 22) radius 1.55
  circle A1 centre (32.373789, 8) radius 1.55
  circle A2 centre (32.373789, 22) radius 3
  circle A3 centre (32.373789, 8) radius 3
  dimension "d323" = 4.4
  dimension "d324" = 8
  dimension "d325" = 14
  dimension "d326" = 3.1
  dimension "d327" = 3.1
  dimension "d328" = 6
  dimension "d329" = 6
  constraint perpendicular L3 L4
  constraint perpendicular L4 L5
  constraint parallel L5 L6
  constraint concentric A0 A2
  constraint concentric A1 A3
  measures "d326" diameter of A0
  measures "d327" diameter of A1
  measures "d328" diameter of A2
  measures "d329" diameter of A3
extrude "Extrude45" cut sketch "Sketch45" against normal blind 28 contours L5 L6 A0 | L5 L6 A0 | A1 picked at (32.867751, 21.095376) picked at (31.731318, 22.805634) picked at (31.590811, 8.423854) bodies 7
extrude "Extrude46" cut sketch "Sketch45" against normal blind 1 contours L5 L6 A0 A2 | L5 L6 A0 A2 | A3 picked at (33.216498, 19.635137) picked at (31.085536, 19.845902) picked at (33.850055, 5.969872) bodies 7
sketch "Sketch46" plane through (119.500002, 0, 0) normal (-1, 0, 0) x (0, -1, 0)
  circle A0 centre (-32.373789, 22) radius 1.55
  circle A1 centre (-32.373789, 8) radius 1.55
  line L0 (-37.687511, 0) -> (-27.973789, 0)
  line L1 (-27.973789, 0) -> (-27.973789, 30)
  line L2 (-27.973789, 30) -> (-37.687511, 30)
  line L3 (-37.687511, 30) -> (-37.687511, 0)
  circle A2 centre (-32.373789, 22) radius 2.6
  circle A3 centre (-32.373789, 8) radius 2.6
  dimension "d334" = 5.2
  dimension "d335" = 5.2
  constraint concentric A0 A2
  constraint concentric A1 A3
  measures "d334" diameter of A2
  measures "d335" diameter of A3
extrude "Extrude47" cut sketch "Sketch46" against normal blind 1 contours A2 | A3 picked at (-30.13924, 21.793825) picked at (-30.13924, 7.793825) bodies 7
move_body "Move3" bodies 7 to x (1, 0, 0) y (0, 0, 1) z (0, -1, 0) at (0, 60.000001, -30.000001)
move_body "Move4" bodies 7 to x (1, 0, 0) y (0, 1, 0) z (0, 0, 1) at (-65, 0, -23)
move_body "Move5" bodies 7 to x (1, 0, 0) y (0, 1, 0) z (0, 0, 1) at (-37.077895, -3.37021, 0.169539)
move_body "Move6" bodies 7 to x (1, 0, 0) y (0, 1, 0) z (0, 0, 1) at (0, -1, 0)
move_body "Move7" bodies 7 to x (1, 0, 0) y (0, 1, 0) z (0, 0, 1) at (0, 0, 0.8)
combine "Combine4" operation add target body 6 tool bodies 7
move_body "Move8" bodies 6 to x (-1, 0, 0) y (0, 1, 0) z (0, 0, -1) at (48, 0, 7.886655)
move_body "Move9" bodies 6 to x (1, 0, 0) y (0, 1, 0) z (0, 0, 1) at (0, 0, 0.1)
sketch "Sketch49" plane through (0, 0, 0) normal (0, 0, 1) x (1, 0, 0)
  line L0 (80, 50) -> (122.5, 50)
  line L1 (122.5, 50) -> (122.5, 25)
  line L2 (122.5, 25) -> (80, 25)
  line L3 (80, 25) -> (80, 50)
  line L4 (80, 37.5) -> (92.5, 37.5)
  circle A0 centre (92.5, 37.5) radius 12.5
  line L5 (122.5, 37.5) -> (110, 37.5)
  circle A1 centre (110, 37.5) radius 12.5
  dimension "d342" = 42.5
  dimension "d343" = 25
  dimension "d344" = 12.5
  dimension "d345" = 25
  dimension "d346" = 12.5
  constraint horizontal L0
  constraint vertical L1
  constraint horizontal L2
  constraint vertical L3
  constraint midpoint L3 L4.start
  constraint perpendicular L3 L4
  constraint coincident L4.end A0.centre
  constraint midpoint L1 L5.start
  constraint perpendicular L1 L5
  constraint coincident L5.end A1.centre
  constraint tangent L2 A1
  measures "d342" distance of L0.start L0.end
  measures "d343" distance of L0.start L2.end
  measures "d344" distance of L4.start L4.end
  measures "d345" diameter of A0
  measures "d346" distance of L5.start L5.end
extrude "Extrude49" add sketch "Sketch49" along normal blind 60 separate body contours L0 A0 A1 | A0 A1 | A0 A1 | A0 A1 | L2 A0 A1 picked at (101.25, 47.128921) picked at (91.688443, 37.5) picked at (116.624256, 36.907022) picked at (100.021776, 37.5) picked at (101.25, 27.871079) makes body 8
shell "Shell5" thickness 2.5 outward yes removed faces 1 at (104.166667, 33.333333, 60) on bodies 8
move_body "Move10" bodies 8 to x (1, 0, 0) y (0, 0, -1) z (0, 1, 0) at (-76.17, 2.489241, 84.510759)
combine "Combine5" operation add target body 6 tool bodies 8
sketch "Sketch52" plane through (0, 0, 32.010759) normal (0, 0, -1) x (1, 0, 0)
  line L0 (23.577893, -55.62979) -> (19.577893, -55.62979)
  line L1 (19.577893, -55.62979) -> (19.577893, -25.62979)
  line L2 (19.577893, -25.62979) -> (23.577893, -25.62979)
  line L3 (23.577893, -25.62979) -> (23.577893, -55.62979)
  line L4 (30.577893, -55.62979) -> (26.577893, -55.62979)
  line L5 (26.577893, -55.62979) -> (26.577893, -25.62979)
  line L6 (26.577893, -25.62979) -> (30.577893, -25.62979)
  line L7 (30.577893, -25.62979) -> (30.577893, -55.62979)
  line L8 (33.83, 0.010759) -> (16.33, 0.010759)
  line L9 (16.33, 0.010759) -> (16.33, -62.489241)
  line L10 (16.33, -62.489241) -> (33.83, -62.489241)
  line L11 (33.83, -62.489241) -> (33.83, 0.010759)
  line L12 (23.577893, -55.62979) -> (23.577893, -62.489241)
  line L13 (23.577893, -62.489241) -> (26.577893, -62.489241)
  line L14 (26.577893, -62.489241) -> (26.577893, 0.010759)
  line L15 (26.577893, 0.010759) -> (23.577893, 0.010759)
  line L16 (23.577893, 0.010759) -> (23.577893, -62.489241)
  constraint perpendicular L10 L12
  constraint horizontal L13
  constraint vertical L14
  constraint horizontal L15
  constraint vertical L16
extrude "Extrude52" cut sketch "Sketch52" against normal blind 25 contours L3 L5 L8 L10 L12 L13 L14 L15 L16 picked at (24.577893, -35.62979) bodies 6
fillet "Fillet13" radius 1.5 2 edges at (23.577893, 1.239241, 57.010759) (26.577893, 1.239241, 57.010759) on bodies 6
fillet "Fillet14" radius 4.5 2 edges at (19.577893, 40.62979, 32.010759) (30.577893, 40.62979, 32.010759) on bodies 6
fillet "Fillet15" radius 13 2 edges at (19.577893, 40.62979, 22.329605) (30.577893, 40.62979, 22.329605) on bodies 6
fillet "Fillet16" radius 1.5 2 edges at (30.934097, 40.62979, 7.986655) (19.22169, 40.62979, 7.986655) on bodies 6
sketch "Sketch53" plane through (0, 0, 7.986655) normal (0, 0, 1) x (-1, 0, 0)
  line L0 (-15.976437, -55.62979) -> (-34.179349, -55.62979)
  line L1 (-34.179349, -55.62979) -> (-34.179349, -25.62979)
  line L2 (-34.179349, -25.62979) -> (-15.976437, -25.62979)
  line L3 (-15.976437, -25.62979) -> (-15.976437, -55.62979)
  circle A0 centre (-41.95, -71.849998) radius 3.25
  circle A1 centre (-8.05, -6.05) radius 3.25
  circle A2 centre (-8.050001, -71.849998) radius 3.25
  circle A3 centre (-41.95, -6.05) radius 3.25
  line L4 (-48, -81.231732) -> (-2, -81.231732)
  line L5 (-2, -81.231732) -> (-2, 0)
  line L6 (-2, 0) -> (-48, 0)
  line L7 (-48, 0) -> (-48, -81.231732)
  line L8 (-8.050001, -71.849998) -> (-15.050001, -71.849998)
  circle A4 centre (-15.050001, -71.849998) radius 1.775
  dimension "d369" = 7
  dimension "d370" = 3.55
  constraint horizontal L8
  measures "d370" diameter of A4
extrude "Extrude53" cut sketch "Sketch53" against normal blind 32 contours A4 picked at (-14.516928, -72.28308) bodies 6
fillet "Fillet17" radius 15 3 edges at (-42, 0, 16) (-42, 8.874983, 35.032464) (-42, 18.067372, 44.224852) on bodies 1
fillet "Fillet18" radius 10.5 2 edges at (-42, 30.869872, 46.482278) (-42, 32.826168, 46.066455) on bodies 1
fillet "Fillet19" radius 20.5 1 edges at (-42, 59.637723, 23.568888) on bodies 1
fillet "Fillet20" radius 6 1 edges at (-42, 74.582285, 21.593812) on bodies 1
fillet "Fillet21" radius 3.5 30 edges at (-65, 0, 6.33729) (-65, 0.35556, 15.921174) (-65, 4.581291, 25.82461) (-65, 9.064535, 34.899738) (-65, 12.734168, 38.891648) (-65, 18.403495, 43.579164) (-65, 24.990055, 45.445508) (-65, 31.796015, 45.646637) (-65, 45.446193, 35.476996) (-65, 59.980859, 24.348196) (-65, 68.161348, 22.442404) (-65, 73.853928, 20.73212) (-65, 78.473335, 8.957784) (-19, 78.473335, 8.957784) (-19, 73.853928, 20.73212) (-19, 68.161348, 22.442404) (-19, 59.980859, 24.348196) (-19, 45.446193, 35.476996) (-19, 31.796015, 45.646637) (-19, 24.990055, 45.445508) (-19, 18.403495, 43.579164) (-19, 12.734168, 38.891648) (-19, 9.064535, 34.899738) (-19, 4.581291, 25.82461) (-19, 0.35556, 15.921174) (-19, 0, 6.33729) (48, 81.231732, 6.486655) (2, 81.231732, 6.486655) (48, 0, 6.486655) (2, 0, 6.486655) on bodies 1 6
fillet "Fillet22" radius 3.5 10 edges at (19.953947, 62.489241, 32.010759) (1.33, 62.489241, 47.010759) (25.08, 62.489241, 62.010759) (48.83, 62.489241, 47.010759) (30.203947, 62.489241, 32.010759) (19.953947, -0.010759, 32.010759) (1.33, -0.010759, 47.010759) (25.08, -0.010759, 62.010759) (48.83, -0.010759, 47.010759) (30.203947, -0.010759, 32.010759) on bodies 6
fillet "Fillet23" radius 3 8 edges at (25, 81.231732, 7.986655) (46.974874, 80.206606, 7.986655) (48, 40.615866, 7.986655) (46.974874, 1.025126, 7.986655) (25, 0, 7.986655) (3.025126, 1.025126, 7.986655) (2, 40.615866, 7.986655) (3.025126, 80.206606, 7.986655) on bodies 6
named bodies: "Body1", "Body2"
